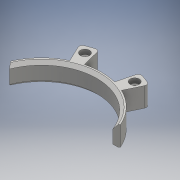
# Autodesk Inventor part: Funnel_Adapter
Saved by Autodesk Inventor 2016 (Build 200138000, 138)
## iProperties
Created: 2015-07-20
Part Number: Funnel_Adapter
Material: Generic
Document SubType Name: Modeling
Designer: bastli
Density: 1 g/cm^3
Appearance: Default
Author: bastli
Autodesk Inventor part; units mm, degrees
ref_plane "YZ Plane" through (0, 0, 0) normal (1, 0, 0) x (0, 1, 0)
ref_plane "XZ Plane" through (0, 0, 0) normal (0, 1, 0) x (-1, 0, 0)
ref_plane "XY Plane" through (0, 0, 0) normal (0, 0, 1) x (1, 0, 0)
derived "Transmission.ipt"
sketch "Sketch1" plane through (0, 0, 0) normal (0, 0, 1) x (1, 0, 0)
  circle A0 centre (-40.963, -23.65) radius 1.55 construction
  circle A1 centre (-30.4039, -36.2339) radius 1.55 construction
  circle A2 centre (-21.0753, -57.9039) radius 1.55 construction
  circle A3 centre (0, -47.3) radius 1.55 construction
  circle A4 centre (16.1776, -44.4475) radius 1.55 construction
  circle A5 centre (39.6086, -47.2037) radius 1.55 construction
  circle A6 centre (40.963, -23.65) radius 1.55 construction
  circle A7 centre (-40.963, 23.65) radius 1.55 construction
  circle A8 centre (-30.4039, 36.2339) radius 1.55 construction
  circle A9 centre (-16.1776, 44.4475) radius 1.55 construction
  circle A10 centre (53.3645, 30.81) radius 1.55 construction
  circle A11 centre (39.6086, 47.2037) radius 1.55 construction
  circle A12 centre (21.0753, 57.9039) radius 1.55 construction
  circle A13 centre (0, 61.62) radius 1.55 construction
  circle A14 centre (0, 47.3) radius 1.55 construction
  circle A15 centre (16.1776, 44.4475) radius 1.55 construction
  circle A16 centre (30.4039, 36.2339) radius 1.55 construction
  circle A17 centre (40.963, 23.65) radius 1.55 construction
  circle A18 centre (-21.0753, 57.9039) radius 1.55 construction
  circle A19 centre (-39.6086, 47.2037) radius 1.55 construction
  circle A20 centre (-53.3645, 30.81) radius 1.55 construction
  circle A21 centre (53.3645, -30.81) radius 1.55 construction
  circle A22 centre (30.4039, -36.2339) radius 1.55 construction
  circle A23 centre (21.0753, -57.9039) radius 1.55 construction
  circle A24 centre (0, -61.62) radius 1.55 construction
  circle A25 centre (-16.1776, -44.4475) radius 1.55 construction
  circle A26 centre (-39.6086, -47.2037) radius 1.55 construction
  circle A27 centre (-53.3645, -30.81) radius 1.55 construction
  circle A28 centre (62.46, 8) radius 2.2 construction
  circle A29 centre (46.46, -8) radius 2.2 construction
  circle A30 centre (-46.46, -8) radius 2.2 construction
  circle A31 centre (-62.46, 8) radius 2.2 construction
  circle A32 centre (-46.46, 8) radius 2.2 construction
  circle A33 centre (-62.46, -8) radius 2.2 construction
  circle A34 centre (46.46, 8) radius 2.2 construction
  circle A35 centre (62.46, -8) radius 2.2 construction
  circle A36 centre (-54.46, 0) radius 7.995 construction
  circle A37 centre (54.46, 0) radius 7.995 construction
  circle A38 centre (0, 0) radius 37.3 construction
  circle A39 centre (0, 0) radius 36 construction
  circle A40 centre (-54.46, 0) radius 21.46 construction
  circle A41 centre (54.46, 0) radius 21.46 construction
  circle A42 centre (-54.46, 0) radius 24.46 construction
  circle A43 centre (54.46, 0) radius 24.46 construction
  circle A44 centre (0, 0) radius 52.46 construction
  line L0 (0, 37.3) -> (0, 52.46) construction
  line L1 (0, 52.46) -> (0, 67.62) construction
  line L2 (0, 0) -> (0, 37.3) construction
  arc A45 (33.6357, 12.8312) -> (-33.6357, 12.8312) centre (0, 0) ccw
  arc A46 (46.9671, 23.3698) -> (-47.0038, 23.2958) centre (0, 0) ccw
  arc A47 (-33.6357, 12.8312) -> (-47.0038, 23.2958) centre (-54.46, 0) ccw
  arc A48 (47.7431, 47.8859) -> (38.8679, 55.3331) centre (0, 0) ccw projected
  arc A49 (-61.2418, -28.669) -> (-65.342, -17.4038) centre (-63.542, -23.1274) ccw projected
  arc A50 (-61.2418, -28.669) -> (-55.4489, -38.7025) centre (0, 0) ccw projected
  arc A51 (-47.7431, -47.8859) -> (-55.4489, -38.7025) centre (-51.7999, -43.4653) ccw projected
  arc A52 (-47.7431, -47.8859) -> (-38.8679, -55.3331) centre (0, 0) ccw projected
  arc A53 (-28.4859, -61.3272) -> (-38.8679, -55.3331) centre (-33.81, -58.5606) ccw projected
  arc A54 (-28.4859, -61.3272) -> (-17.5989, -65.2897) centre (0, 0) ccw projected
  arc A55 (-5.7928, -67.3714) -> (-17.5989, -65.2897) centre (-11.7421, -66.5927) ccw projected
  arc A56 (-5.7928, -67.3714) -> (5.7928, -67.3714) centre (0, 0) ccw projected
  arc A57 (17.5989, -65.2897) -> (5.7928, -67.3714) centre (11.7421, -66.5927) ccw projected
  arc A58 (17.5989, -65.2897) -> (28.4859, -61.3272) centre (0, 0) ccw projected
  arc A59 (38.8679, -55.3331) -> (28.4859, -61.3272) centre (33.81, -58.5606) ccw projected
  arc A60 (38.8679, -55.3331) -> (47.7431, -47.8859) centre (0, 0) ccw projected
  arc A61 (55.4489, -38.7025) -> (47.7431, -47.8859) centre (51.7999, -43.4653) ccw projected
  arc A62 (55.4489, -38.7025) -> (61.2418, -28.669) centre (0, 0) ccw projected
  arc A63 (65.342, -17.4038) -> (61.2418, -28.669) centre (63.542, -23.1274) ccw projected
  arc A64 (65.342, -17.4038) -> (65.342, 17.4038) centre (0, 0) ccw projected
  arc A65 (61.2418, 28.669) -> (65.342, 17.4038) centre (63.542, 23.1274) ccw projected
  arc A66 (61.2418, 28.669) -> (55.4489, 38.7025) centre (0, 0) ccw projected
  arc A67 (47.7431, 47.8859) -> (55.4489, 38.7025) centre (51.7999, 43.4653) ccw projected
  arc A68 (28.4859, 61.3272) -> (38.8679, 55.3331) centre (33.81, 58.5606) ccw projected
  arc A69 (28.4859, 61.3272) -> (17.5989, 65.2897) centre (0, 0) ccw projected
  arc A70 (5.7928, 67.3714) -> (17.5989, 65.2897) centre (11.7421, 66.5927) ccw projected
  arc A71 (-17.5989, 65.2897) -> (-5.7928, 67.3714) centre (-11.7421, 66.5927) ccw projected
  arc A72 (-17.5989, 65.2897) -> (-28.4859, 61.3272) centre (0, 0) ccw projected
  arc A73 (-38.8679, 55.3331) -> (-28.4859, 61.3272) centre (-33.81, 58.5606) ccw projected
  arc A74 (-38.8679, 55.3331) -> (-47.7431, 47.8859) centre (0, 0) ccw projected
  arc A75 (-55.4489, 38.7025) -> (-47.7431, 47.8859) centre (-51.7999, 43.4653) ccw projected
  arc A76 (-55.4489, 38.7025) -> (-61.2418, 28.669) centre (0, 0) ccw projected
  arc A77 (-65.342, 17.4038) -> (-61.2418, 28.669) centre (-63.542, 23.1274) ccw projected
  arc A78 (-65.342, 17.4038) -> (-65.342, -17.4038) centre (0, 0) ccw projected
  arc A79 (5.7928, 67.3714) -> (-5.7928, 67.3714) centre (0, 0) ccw projected
  circle A80 centre (-42.275, 30.6584) radius 1.05 projected
  circle A81 centre (-48.7495, 30.0833) radius 1.05 projected
  circle A82 centre (42.275, -30.6584) radius 1.05 projected
  circle A83 centre (48.7495, -30.0833) radius 1.05 projected
  arc A84 (35.7014, 15.6974) -> (-35.7014, 15.6974) centre (0, 0) ccw
  line L3 (-16.7649, 35.2128) -> (-22.5509, 47.3657)
  line L4 (-9.7917, 37.7508) -> (-13.1711, 50.7797)
  arc A85 (46.992, 23.2921) -> (33.6357, 12.8312) centre (54.46, 0) ccw
  line L5 (9.7917, 37.7508) -> (13.1711, 50.7797)
  line L6 (22.5509, 47.3657) -> (16.7649, 35.2128)
  point P0 (0, 61.62)
  point P1 (0, 47.3)
  point P2 (-39.6086, 47.2037)
  point P3 (-30.4039, 36.2339)
  point P4 (39.6086, 47.2037)
  point P5 (30.4039, 36.2339)
  point P6 (30.4039, -36.2339)
  point P7 (39.6086, -47.2037)
  point P8 (0, -47.3)
  point P9 (0, -61.62)
  point P10 (-39.6086, -47.2037)
  point P11 (-30.4039, -36.2339)
  point P12 (0, 0)
  point P13 (0, 0)
  dimension "d0" = 72
  dimension "d3" = 42.92
  dimension "d4" = 42.92
  dimension "d6" = 3
  dimension "d7" = 3
  dimension "d33" = 3
  dimension "d34" = 4.5
  dimension "d35" = 4.5
  dimension "d36" = 4.5
  dimension "d37" = 4.5
  constraints: 29 point on circle, 21 coincident, 14 end point, 9 centre point, 4 line through centre, 2 vertical, 1 collinear, 1 point on line, 1 vertical alignment, 7 other
  measures "d3" diameter of A40
  measures "d4" diameter of A41
  measures "d6" radial gap between concentric circles of A40 A42
  measures "d34" distance from line of L4 A9.centre
  measures "d35" distance from line of L3 A9.centre
  measures "d36" distance from line of A15.centre L5
  measures "d37" distance from line of L6 A15.centre
extrude "Extrusion1" add sketch "Sketch1" along normal blind 12.7 contours A45 A47 A84 A85 | A84 L5 A46 L6 | L3 A46 L4 A84
sketch "Sketch2" plane through (0, 0, 12.7) normal (0, 0, 1) x (1, 0, 0)
  circle A0 centre (-30.4039, 36.2339) radius 1.55 projected
  circle A1 centre (-16.1776, 44.4475) radius 1.55 projected
  circle A2 centre (0, 47.3) radius 1.55 projected
  circle A3 centre (16.1776, 44.4475) radius 1.55 projected
  circle A4 centre (30.4039, 36.2339) radius 1.55 projected
  point P0 (0, 0)
  constraints: 5 coincident
hole "Hole1" at (-30.4039, 36.2339, 12.7) at (0, 47.3, 12.7) at (30.4039, 36.2339, 12.7) at (16.1776, 44.4475, 12.7) at (-16.1776, 44.4475, 12.7) direction (0, 0, -1) diameter 3.1 end through all
hole "Hole2" at (-30.4039, 36.2339, 12.7) at (-16.1776, 44.4475, 12.7) at (0, 47.3, 12.7) at (16.1776, 44.4475, 12.7) at (30.4039, 36.2339, 12.7) direction (0, 0, -1) diameter 6 depth 3
chamfer "Chamfer1" distance 2 angle 45 1 edges at (0, 36, 0)
chamfer "Chamfer2" distance 2 angle 45 1 edges at (0, 36, 12.7)
fillet "Fillet1" radius 2 4 edges at (22.5509, 47.3657, 6.35) (13.1711, 50.7797, 6.35) (-13.1711, 50.7797, 6.35) (-22.5509, 47.3657, 6.35)
equation "\"d0\" = funnel_width"
equation "\"d3\" = d5"
equation "\"d4\" = d5"
equation "\"d7\" = thickness"
equation "\"d33\" = thickness"
equation "\"d34\" = 1.5 * thickness"
equation "\"d35\" = 1.5 * thickness"
equation "\"d36\" = 1.5 * thickness"
equation "\"d37\" = 1.5 * thickness"
equation "\"funnel_width\" = 72"
equation "\"thickness\" = 3"
equation "\"d5\" = 42.92"
body "Solid1"
